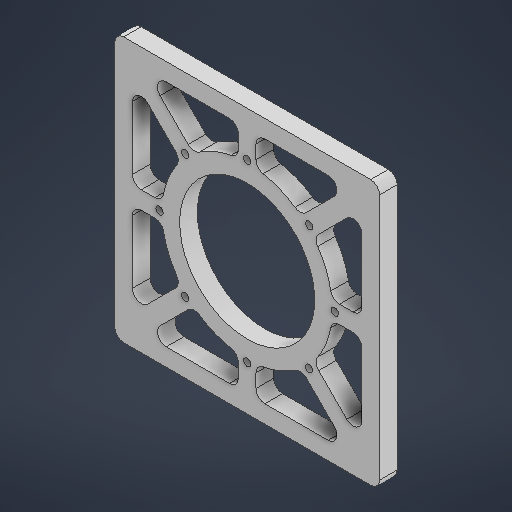
# Autodesk Inventor part: Aufhängung_Front_Koppeltest
Saved by Autodesk Inventor 2027 (Build 310192060, 192F)
## iProperties
Created: 2016-02-20
Part Number: Aufhängung_Front_Koppeltest
Material: Generisch
Document SubType Name: Modeling
Designer: Halle20
Density: 1 g/cm^3
Appearance: Vorgabe
Author: Halle20
Autodesk Inventor part; units mm, degrees
ref_plane "YZ Plane" through (0, 0, 0) normal (1, 0, 0) x (0, 1, 0)
ref_plane "XZ Plane" through (0, 0, 0) normal (0, 1, 0) x (-1, 0, 0)
ref_plane "XY Plane" through (0, 0, 0) normal (0, 0, 1) x (1, 0, 0)
sketch "Sketch5" plane through (0, 0, 0) normal (0, 0, 1) x (1, 0, 0)
  line L0 (0, 0) -> (300, 0)
  line L1 (300, 0) -> (300, 500)
  line L2 (300, 500) -> (0, 500)
  line L3 (0, 500) -> (0, 0)
  line L4 (20, 480) -> (280, 480)
  line L5 (280, 480) -> (280, 20)
  line L6 (280, 20) -> (20, 20)
  line L7 (20, 20) -> (20, 480)
  circle A0 centre (150, 250) radius 90
  circle A1 centre (150, 250) radius 76.5
  line L8 (20, 240) -> (280, 240)
  line L9 (280, 240) -> (280, 260)
  line L10 (280, 260) -> (20, 260)
  line L11 (20, 260) -> (20, 240)
  line L12 (140, 20) -> (160, 20)
  line L13 (160, 20) -> (160, 480)
  line L14 (160, 480) -> (140, 480)
  line L15 (140, 480) -> (140, 20)
  line L16 (150, 250) -> (333.8478, 250) construction
  line L17 (12.9289, 127.0711) -> (287.0711, 401.2132)
  line L18 (287.0711, 372.9289) -> (12.9289, 98.7868)
  line L19 (150, 250) -> (333.8478, 250) construction
  line L20 (12.9289, 372.9289) -> (287.0711, 98.7868)
  line L21 (287.0711, 127.0711) -> (12.9289, 401.2132)
  line L22 (150, 250) -> (79.7843, 179.7843)
  circle A2 centre (150, 250) radius 96.5
  line L23 (0, 100) -> (300, 100)
  line L24 (0, 400) -> (300, 400)
  line L25 (0, 120) -> (300, 120)
  line L26 (0, 380) -> (300, 380)
  point P0 (150, 150.7)
  point P1 (220.2157, 179.7843)
  point P2 (249.3, 250)
  point P3 (220.2157, 320.2157)
  point P4 (150, 349.3)
  point P5 (79.7843, 320.2157)
  point P6 (50.7, 250)
  point P7 (60.5573, 240)
  point P8 (79.6834, 193.8255)
  point P9 (20, 134.1421)
  point P10 (160, 339.4427)
  point P11 (280, 394.1421)
  point P12 (206.1745, 320.3166)
  point P13 (239.4427, 260)
  point P14 (220.3166, 306.1745)
  point P15 (280, 365.8579)
  point P16 (93.8255, 179.6834)
  point P17 (140, 160.5573)
  point P18 (20, 105.8579)
  point P19 (140, 339.4427)
  point P20 (93.8255, 320.3166)
  point P21 (20, 394.1421)
  point P22 (220.3166, 193.8255)
  point P23 (239.4427, 240)
  point P24 (280, 134.1421)
  point P25 (160, 160.5573)
  point P26 (206.1745, 179.6834)
  point P27 (280, 105.8579)
  point P28 (79.6834, 306.1745)
  point P29 (60.5573, 260)
  point P30 (20, 365.8579)
  point P31 (54.0195, 240)
  point P32 (75.0605, 189.2026)
  point P33 (89.2026, 175.0605)
  point P34 (140, 154.0195)
  point P35 (75.0605, 310.7974)
  point P36 (54.0195, 260)
  point P37 (140, 345.9805)
  point P38 (89.2026, 324.9395)
  point P39 (210.7974, 324.9395)
  point P40 (160, 345.9805)
  point P41 (245.9805, 260)
  point P42 (224.9395, 310.7974)
  point P43 (224.9395, 189.2026)
  point P44 (245.9805, 240)
  point P45 (160, 154.0195)
  point P46 (210.7974, 175.0605)
  point P47 (34.1421, 380)
  point P48 (140, 380)
  point P49 (160, 380)
  point P50 (265.8579, 380)
  point P51 (140, 120)
  point P52 (34.1421, 120)
  point P53 (265.8579, 120)
  point P54 (160, 120)
  dimension "d28" = 300
  dimension "d29" = 500
  dimension "d30" = 20
  dimension "d62" = 180
  dimension "d63" = 153
  dimension "d84" = 20
  dimension "d85" = 20
  dimension "d92" = 99.3
  dimension "d98" = 20
  dimension "d104" = 20
  dimension "d105" = 20
  constraints: 54 end point, 11 parallel, 8 point on line, 6 perpendicular, 5 horizontal, 3 centre point, 1 coincident, 3 other
  measures "d28" distance of L2.end L1.end
  measures "d29" distance of L1.end L0.end
  measures "d30" distance between parallel lines of L2 L4
  measures "d62" diameter of A0
  measures "d63" diameter of A1
  measures "d84" distance of L9.end L8.end
  measures "d85" distance of L14.end L13.end
  measures "d92" distance of L16.start L22.end
  measures "d98" radial gap between concentric circles of A1 A2
  measures "d104" distance between parallel lines of L23 L25
  measures "d105" distance between parallel lines of L24 L26
extrude "Extrusion5" add sketch "Sketch5" along normal blind 20 contours L3 L25 L7 L18 L23 | L23 L20 L5 L25 L1 | L3 L26 L7 L25 | L18 L7 L23 | L25 L5 L26 L1 | L23 L5 L20 | L3 L24 L21 L7 L26 | L25 L18 L7 | L7 L17 A2 L18 L25 | L18 L25 L15 L23 L7 | L26 L5 L17 L24 L1 | L25 L20 A2 L21 L5 | L5 L20 L25 | L5 L23 L13 L25 L20 | L26 L21 A2 L20 L7 | L7 L21 L26 | L15 L25 L13 L23 | L26 L17 L5 | L5 L18 A2 L17 L26 | L24 L7 L21 | L7 L24 L15 L26 L21 | L7 L10 A2 L8 | A2 L8 A0 L17 | L17 A0 L22 A2 | A2 L22 A0 L18 | L18 A0 L15 A2 | L15 A2 L13 L25 | L17 L5 L24 | L17 L26 L13 L24 L5 | L8 A2 L10 L5 | A2 L20 A0 L21 | L21 A0 L8 A2 | A2 L13 A0 L20 | A2 L21 A0 L20 | L20 A0 L10 A2 | A2 L15 A0 L21 | L26 L13 A2 L15 | L15 L24 L13 L26 | A2 L10 A0 L8 | L17 A1 L22 A0 | A0 L8 A1 L17 | L18 A1 L15 A0 | A0 L22 A1 L18 | L15 A0 L13 A2 | A2 L10 A0 L18 | L18 A0 L17 A2 | L17 A0 L13 A2 | L8 A0 L10 A2 | L21 A1 L8 A0 | A0 L20 A1 L21 | A0 L13 A1 L20 | L20 A1 L10 A0 | A0 L21 A1 L20 | A0 L15 A1 L21 | A2 L13 A0 L15 | A0 L10 A1 L8 | L15 A1 L13 A0 | L18 A1 L17 A0 | A0 L10 A1 L18 | L17 A1 L13 A0 | L8 A1 L10 A0 | A0 L13 A1 L15
fillet "Fillet1" radius 10 32 edges at (160, 154.0195, 10) (160, 120, 10) (265.8579, 120, 10) (280, 134.1421, 10) (210.7974, 175.0605, 10) (224.9395, 189.2026, 10) (245.9805, 240, 10) (280, 240, 10) (280, 260, 10) (245.9805, 260, 10) (224.9395, 310.7974, 10) (280, 365.8579, 10) (265.8579, 380, 10) (210.7974, 324.9395, 10) (160, 345.9805, 10) (160, 380, 10) (140, 380, 10) (140, 345.9805, 10) (34.1421, 380, 10) (89.2026, 324.9395, 10) (75.0605, 310.7974, 10) (20, 365.8579, 10) (20, 240, 10) (20, 260, 10) (54.0195, 260, 10) (54.0195, 240, 10) (75.0605, 189.2026, 10) (89.2026, 175.0605, 10) (20, 134.1421, 10) (34.1421, 120, 10) (140, 120, 10) (140, 154.0195, 10)
sketch "Sketch6" plane through (300, 10, 0) normal (1, 0, 0) x (0, 0, -1)
  line L0 (0, 0) -> (-20, 0) projected
  line L1 (-10, 0) -> (-10, 480)
  line L2 (0, 480) -> (-20, 480) projected
  line L3 (-10, 240) -> (-10, 120)
  line L4 (-10, 120) -> (-10, 360)
  point P0 (0, -10)
  dimension "d53" = 120
  dimension "d54" = 240
  constraints: 6 end point, 3 midpoint, 2 point on line
  measures "d53" distance of L3.start L3.end
  measures "d54" distance of L3.end L4.end
hole "Hole2" at (300, 130, 10) at (300, 250, 10) at (300, 370, 10) direction (-1, 0, 0) diameter 3.2 depth 20 tip angle 118 clearance for "Socket Head Cap Screw ISO 4762" size "M3" standard "ISO"
hole "Hole3" at (79.7843, 179.7843, 0) direction (0, 0, 1) diameter 8.376 end through all thread size "M10x1.5" class "6H" standard "ISO Metric profile"
fillet "Fillet2" radius 10 4 edges at (0, 100, 10) (0, 400, 10) (300, 400, 10) (300, 100, 10)
pattern_circular "Circular Pattern1" count 8 over 360 about axis through (150, 250, 0) along (0, 0, 1) of "Hole3"
body "Solid3"
